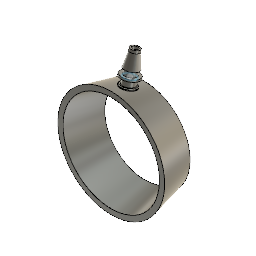
Pneumotach_Filter_V1 (Autodesk Fusion 360 design; units mm, degrees)
Autodesk Fusion 360 part; units mm, degrees
sketch "Sketch1" plane through (0, 0, 0) normal (1, 0, 0) x (0, 1, 0)
  line L0 (3, 0) -> (3, 17.5)
  line L1 (14, 0) -> (14, 14.85)
  line L2 (3, 17.5) -> (14, 14.85)
  line L3 (3, 17.5) -> (3, 15.75)
  line L4 (3, 17.5) -> (3, 15.85)
  line L5 (14, 14.85) -> (14, 13.05)
  line L6 (3, 15.75) -> (14, 13.05)
  dimension "d1" = 17.5
  dimension "d2" = 14.85
  dimension "d4" = 1.65
  dimension "d5" = 1.8
  constraint vertical L0
  constraint vertical L1
  constraint parallel L0 L3
  constraint parallel L0 L4
  constraint parallel L1 L5
  measures "d1" distance of L0.start L0.end
  measures "d2" distance of L1.start L1.end
  measures "d4" distance of L0.end L4.end
  measures "d5" distance of L1.end L5.end
revolve "Revolve1" add sketch "Sketch1" angle 360 about axis through (0, 1.75, 0) along (0, 1, 0) makes body 1
ref_plane "WorkPlane1" through (0, 8.5, 16.175) normal (0, 0.234209, 0.972186) x (-1, 0, 0)
sketch "Sketch2" plane through (0, 8.5, 16.175) normal (0, 0.234209, 0.972186) x (-1, 0, 0)
  circle A0 centre (0, 0) radius 1.9
  dimension "d8" = 3.8
  constraint coincident A0.centre origin
  measures "d8" diameter of A0
extrude "Extrude1" add sketch "Sketch2" along normal blind 2.5 separate body makes body 2
sketch "Sketch3" plane through (0, 4.7347, 19.6536) normal (0, 0.234209, 0.972186) x (-1, 0, 0)
  circle A0 centre (0, -4.4753) radius 1.9
sketch "Sketch4" plane through (0, 9.0855, 18.6055) normal (0, 0.234209, 0.972186) x (1, 0, 0)
  circle A0 centre (0, 0) radius 2.9
  dimension "d11" = 5.8
  constraint coincident A0.centre origin
  measures "d11" diameter of A0
extrude "Extrude2" add sketch "Sketch4" along normal blind 0.6 and the other way blind 0 bodies 2
sketch "Sketch5" plane through (0, 4.7347, 19.6536) normal (0, 0.234209, 0.972186) x (1, 0, 0)
  circle A0 centre (0, 4.5) radius 1.9
  dimension "d16" = 3.8
  measures "d16" diameter of A0
ref_plane "WorkPlane2" through (0, 9.226, 19.1888) normal (0, 0.234209, 0.972186) x (1, 0, 0)
sketch "Sketch6" plane through (0, 9.226, 19.1888) normal (0, 0.234209, 0.972186) x (1, 0, 0)
  circle A0 centre (0, 0) radius 1.9
  dimension "d18" = 3.8
  constraint coincident A0.centre origin
  measures "d18" diameter of A0
extrude "Extrude3" add sketch "Sketch6" along normal blind 1.6 bodies 2
ref_plane "WorkPlane3" through (0, 9.6008, 20.7443) normal (0, 0.234209, 0.972186) x (1, 0, 0)
sketch "Sketch7" plane through (0, 9.6008, 20.7443) normal (0, 0.234209, 0.972186) x (1, 0, 0)
ref_plane "WorkPlane4" through (1.9, 9.4912, 20.2893) normal (1, 0, 0) x (0, -0.972186, 0.234209)
ref_plane "WorkPlane5" through (0, 9.4912, 20.2893) normal (1, 0, 0) x (0, -0.972186, 0.234209)
sketch "Sketch8" plane through (0, 9.4912, 20.2893) normal (1, 0, 0) x (0, 1, 0)
ref_plane "WorkPlane6" through (0, 9.4912, 20.2893) normal (1, 0, 0) x (0, -0.972186, 0.234209)
sketch "Sketch9" plane through (0, 9.4912, 20.2893) normal (1, 0, 0) x (0, 1, 0)
  line L0 (2.5859, 4.4366) -> (2.3273, -0.0695)
  line L1 (2.0742, 4.5594) -> (1.3553, 0.1637)
  line L2 (2.0742, 4.5594) -> (2.5859, 4.4366)
  line L3 (1.3553, 0.1637) -> (2.3273, -0.0695)
  constraint parallel L2 L3
revolve "Revolve2" add sketch "Sketch9" angle 360 about axis through (0, 9.226, 19.1888) along (0, -0.234209, -0.972186) separate body makes body 3
ref_plane "WorkPlane7" through (0, 10.749, 25.405) normal (0, 0.234209, 0.972186) x (1, 0, 0)
sketch "Sketch10" plane through (0, 10.749, 25.405) normal (0, 0.234209, 0.972186) x (1, 0, 0)
  circle A0 centre (0, 0) radius 0.949
  circle A1 centre (0, 0) radius 1.475
  dimension "d29" = 1.898
  dimension "d30" = 2.95
  constraint coincident A0.centre A1.centre
  constraint concentric A0 A1
  measures "d29" diameter of A0
  measures "d30" diameter of A1
extrude "Extrude4" add sketch "Sketch10" along normal blind 0.5 and the other way blind 0.4 bodies 3
hole "Hole1" at (0, 9.6008, 20.7443) direction (0, -0.234209, -0.972186) diameter 2.5 depth 8 tip angle 180 bodies 1 2
sketch "Sketch11" plane through (0, 4.1492, 17.2231) normal (0, -0.234209, -0.972186) x (1, 0, 0)
  circle A0 centre (0, -4.4753) radius 1.25
  circle A1 centre (0, -4.4753) radius 1.9
  circle A2 centre (0, -4.4753) radius 2.5149
  circle A3 centre (0, -4.4753) radius 1.9
  constraint concentric A0 A2
  constraint concentric A2 A3
extrude "Extrude5" add sketch "Sketch11" against normal blind 0.5 contours A2 bodies 2 1
fillet "Fillet2" radius 0.25 1 edges at (-2.3447, 7.733, 16.8741) on bodies 2
